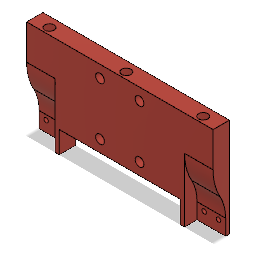
X-carriage-III-part1-rev1_microswitch2 v5 (Autodesk Fusion 360 design; units mm, degrees)
Autodesk Fusion 360 part; units mm, degrees
box "BoxPrimitive1" add length 7.5 width 85 height 45 placed x (0, 0, -1) y (-1, 0, 0) z (0, 1, 0) at (100, 0, 30)
move_body "Move1" bodies 1 to x (1, 0, 0) y (0, 1, 0) z (0, 0, 1) at (-60, 0, -30)
move_body "Move2" bodies 1 to x (1, 0, 0) y (0, 1, 0) z (0, 0, 1) at (2.5, 0, 0)
sketch "Sketch4" plane through (0, 45, 0) normal (0, 1, 0) x (-1, 0, 0)
  line L0 (-42.5, -7.5) -> (42.5, -7.5)
  line L1 (42.5, -7.5) -> (42.5, 0)
  line L2 (42.5, 0) -> (-42.5, 0)
  line L3 (-42.5, 0) -> (-42.5, -7.5)
  circle A0 centre (-35, -3) radius 2.1
  circle A1 centre (-17.5, -3) radius 2.1
  circle A2 centre (0, -3) radius 2.1
  circle A3 centre (17.5, -3) radius 2.1
  circle A4 centre (35, -3) radius 2.1
  line L4 (42.5, -3) -> (-42.5, -3) construction
  line L5 (0, 0) -> (0, -12) construction
  dimension "d13" = 4.2
  dimension "d14" = 4.2
  dimension "d15" = 4.2
  dimension "d16" = 4.2
  dimension "d17" = 4.2
  dimension "d18" = 17.5
  dimension "d19" = 17.5
  dimension "d20" = 17.5
  dimension "d21" = 17.5
  dimension "d27" = 3
  measures "d13" diameter of A0
  measures "d14" diameter of A1
  measures "d15" diameter of A2
  measures "d16" diameter of A3
  measures "d17" diameter of A4
  measures "d27" distance of L5.start
extrude "Extrude2" cut sketch "Sketch4" against normal blind 8 contours A0 | A2 | A4
sketch "Sketch5" plane through (0, 0, 0) normal (0, 0, 1) x (1, 0, 0)
  line L0 (-42.5, 45) -> (-42.5, 0)
  line L1 (-42.5, 0) -> (42.5, 0)
  line L2 (42.5, 0) -> (42.5, 45)
  line L3 (42.5, 45) -> (-42.5, 45)
  circle A0 centre (-9, 39.5) radius 2
  circle A1 centre (9, 39.5) radius 2
  circle A2 centre (-9, 15.5) radius 2
  circle A3 centre (9, 15.5) radius 2
  line L4 (-9, 39.5) -> (9, 39.5)
  line L5 (9, 39.5) -> (9, 15.5)
  line L6 (9, 15.5) -> (-9, 15.5)
  line L7 (-9, 15.5) -> (-9, 39.5)
  circle A4 centre (9, 39.5) radius 3.75
  circle A5 centre (-9, 39.5) radius 3.75
  circle A6 centre (9, 15.5) radius 3.75
  circle A7 centre (-9, 15.5) radius 3.75
  dimension "d38" = 4
  dimension "d39" = 4
  dimension "d40" = 4
  dimension "d41" = 4
  dimension "d42" = 18
  dimension "d43" = 18
  dimension "d44" = 24
  dimension "d45" = 24
  dimension "d52" = 7.5
  dimension "d53" = 7.5
  dimension "d54" = 7.5
  dimension "d55" = 7.5
  dimension "d97" = 5.5
  dimension "d98" = 9
  measures "d38" diameter of A0
  measures "d39" diameter of A1
  measures "d40" diameter of A3
  measures "d41" diameter of A2
  measures "d52" diameter of A4
  measures "d53" diameter of A5
  measures "d54" diameter of A6
  measures "d55" diameter of A7
  measures "d97" distance of origin
  measures "d98" distance of origin
extrude "Extrude7" cut sketch "Sketch5" against normal through all contours A0 L4 L7 | A0 L4 L7
extrude "Extrude8" cut sketch "Sketch5" against normal through all contours A1 L4 L5 | A1 L4 L5
extrude "Extrude9" cut sketch "Sketch5" against normal through all contours A3 L5 L6 | A3 L5 L6
extrude "Extrude10" cut sketch "Sketch5" against normal through all contours A2 L6 L7 | A2 L6 L7
extrude "Extrude11" cut sketch "Sketch5" along normal blind 4 from surface at -7.5 contours A0 L4 L7 A5 | A0 L4 L7 A5 | A1 L4 L5 A4 | A1 L4 L5 A4 | A2 L6 L7 A7 | A2 L6 L7 A7 | A3 L5 L6 A6 | A3 L5 L6 A6
move_body "Move3" bodies 1 to x (1, 0, 0) y (0, 1, 0) z (0, 0, 1) at (0, -27.5, 0)
sketch "Sketch10" plane through (42.5, 0, 0) normal (1, 0, 0) x (0, 0, -1)
  line L0 (7.5, -27.5) -> (1.8, -27.5)
  line L1 (1.8, -27.5) -> (1.8, -15)
  line L2 (1.8, -15) -> (7.5, -15) construction
  line L3 (7.5, -15) -> (7.5, -27.5)
  line L4 (1.8, -15) -> (7.5, -5)
  line L5 (7.5, -5) -> (7.5, -27.5)
  line L6 (0, -27.5) -> (5.7, -27.5)
  line L7 (5.7, -27.5) -> (5.7, -15)
  line L8 (5.7, -15) -> (0, -15)
  line L9 (0, -15) -> (0, -27.5)
  line L10 (0, 17.5) -> (0, -27.5)
  line L11 (5.7, -15) -> (0, -5)
  dimension "d99" = 5.7
  dimension "d100" = 12.5
  dimension "d102" = 10
  dimension "d121" = 5.7
  dimension "d122" = 10
  measures "d121" distance of origin
extrude "Extrude14" cut sketch "Sketch10" against normal blind 13 contours L0 L1 L6 L7 L8 | L1 L6 L8 L9 L10 | L4 L8 L11 | L4 L8 L10 L11
fillet "Fillet3" radius 20 1 edges at (36, -15, -5.7)
fillet "Fillet4" radius 25 1 edges at (36, -5, 0)
sketch "Sketch11" plane through (0, 0, -7.5) normal (0, 0, -1) x (-1, 0, 0)
  line L0 (-32.75, -22.5) -> (-39.25, -22.5) construction
  circle A0 centre (-39.25, -22.5) radius 1
  circle A1 centre (-32.75, -22.5) radius 1
  line L1 (-29.5, -27.5) -> (-42.5, -27.5)
  line L2 (-36, -22.5) -> (-36, -27.5) construction
  circle A2 centre (-9, 12) radius 3.75
  circle A3 centre (9, -12) radius 3.75
  circle A4 centre (9, 12) radius 3.75
  circle A5 centre (-9, -12) radius 3.75
  line L3 (-42.5, 17.5) -> (-42.5, -27.5)
  line L4 (-42.5, -27.5) -> (42.5, -27.5)
  line L5 (42.5, -27.5) -> (42.5, 17.5)
  line L6 (42.5, 17.5) -> (-42.5, 17.5)
  dimension "d110" = 6.5
  dimension "d111" = 2
  dimension "d112" = 2
  dimension "d113" = 5
  measures "d111" diameter of A0
  measures "d112" diameter of A1
  measures "d113" distance of L0 L1
extrude "Extrude15" cut sketch "Sketch11" against normal through all contours A0 | A1
mirror "Mirror3" about plane through (0, 0, 0) normal (1, 0, 0) of "Extrude14", "Fillet3", "Fillet4", "Extrude15"
sketch "Sketch13" plane through (0, 0, -7.5) normal (0, 0, -1) x (-1, 0, 0)
  line L0 (-27.5, -17.5) -> (27.5, -17.5)
  line L1 (27.5, -17.5) -> (27.5, -27.5)
  line L2 (27.5, -27.5) -> (-27.5, -27.5)
  line L3 (-27.5, -27.5) -> (-27.5, -17.5)
  line L4 (42.5, -27.5) -> (-42.5, -27.5)
  dimension "d118" = 55
  dimension "d119" = 10
  measures "d119" distance of origin
extrude "Extrude16" cut sketch "Sketch13" against normal through all
sketch "Sketch15" plane through (0, -17.5, 0) normal (0, -1, 0) x (1, 0, 0)
  line L0 (27.5, 0) -> (-27.5, 0)
  line L1 (-27.5, 0) -> (-27.5, -7.5)
  line L2 (-27.5, -7.5) -> (27.5, -7.5)
  line L3 (27.5, -7.5) -> (27.5, 0)
  circle A0 centre (-17.5, -3) radius 2.1
  circle A1 centre (17.5, -3) radius 2.1
  line L4 (-17.5, -3) -> (17.5, -3) construction
  dimension "d129" = 4.2
  dimension "d130" = 4.2
  dimension "d131" = 35
  dimension "d132" = 17.5
  dimension "d134" = 3
  measures "d129" diameter of A0
  measures "d130" diameter of A1
  measures "d132" distance of origin
  measures "d134" distance of origin L4
extrude "Extrude17" cut sketch "Sketch15" against normal blind 8 contours A0 | A1
equation "d132 = ( 35 / 2 ) * 1 mm"
